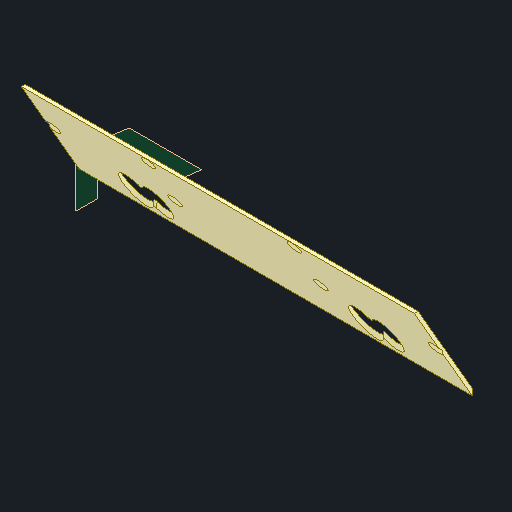
# Autodesk Inventor part: front
Saved by Autodesk Inventor 2023 (Build 270158000, 158)
## iProperties
Created: 2024-05-26
Part Number: front
Material: Nylon 6
Document SubType Name: Modeling
Designer: szymo
Density: 1.12 g/cm^3
Appearance: Nylon 6
Mass: 13.8387 g
Surface Area: 179.282 cm^2
Volume: 12.3559 cm^3
Author: szymo
Autodesk Inventor part; units mm, degrees
ref_plane "YZ Plane" through (0, 0, 0) normal (1, 0, 0) x (0, 1, 0)
ref_plane "XZ Plane" through (0, 0, 0) normal (0, 1, 0) x (-1, 0, 0)
ref_plane "XY Plane" through (0, 0, 0) normal (0, 0, 1) x (1, 0, 0)
ref_plane "Work Plane1" through (-178, 0.5, -3.5) normal (-1, 0, 0) x (0, 0, 1)
sketch "Sketch1" plane through (-178, 0.5, -3.5) normal (-1, 0, 0) x (0, 0, 1)
  line L0 (3.5, 3.5) -> (-1, 3.5) projected
  line L1 (-1, 3.5) -> (-1, -0.5) projected
  line L2 (-1, -0.5) -> (-4.5, -0.5) projected
  line L3 (-4.5, -0.5) -> (-4.5, -14.5) projected
  line L4 (-4.5, -14.5) -> (4.5, -0.5) projected
  line L5 (4.5, -0.5) -> (3.5, -0.5) projected
  line L6 (3.5, -0.5) -> (3.5, 3.5) projected
  circle A0 centre (8.5, 158.5) radius 3 projected
  circle A1 centre (8.5, 158.5) radius 25
  circle A2 centre (13, 116) radius 15 projected
  line L7 (3.5, 3.5) -> (28, 45.9352)
  line L8 (3.5, 0.5) -> (29.7321, 45.9352)
  line L9 (29.7321, 45.9352) -> (28, 45.9352)
  line L10 (28, 45.9352) -> (28, 131) projected
  dimension "d0" = 50
  dimension "d1" = 30
  dimension "d3" = 1.5
  dimension "d4" = 3
  dimension "d5" = 1.7321
  constraints: 6 end point, 2 point on line, 1 centre point, 1 coincident, 1 horizontal, 1 parallel
  measures "d0" diameter of A1
  measures "d1" angle of L7 L6
  measures "d3" distance between parallel lines of L8 L7
  measures "d4" distance of L8.start L0.start
  measures "d5" distance of L7.end L8.end
ref_plane "Work Plane2" through (0, -14, -8) normal (1, 0, 0) x (0, 1, 0)
extrude "Extrusion1" add sketch "Sketch1" against normal up to surface (178 mm away) contours L7 L9 L8 L6
ref_plane "Work Plane3" through (-141.1151, 26.996, 4.2847) normal (0, -0.9925462, 0.1218693) x (1, 0, 0)
sketch "Sketch3" plane through (-141.1151, 26.996, 4.2847) normal (0, -0.9925462, 0.1218693) x (1, 0, 0)
  line L0 (89.3087, 5.4518) -> (89.3087, -5.4534)
  spline S0 degree 3 poles (89.3087, -5.4534) (89.308, -5.5772) (89.3587, -5.6989) (89.4451, -5.7853) (89.4649, -5.8051) (89.4865, -5.823) (89.5096, -5.8388) (89.529, -5.8521) (89.5494, -5.864) (89.5707, -5.8743) (89.5866, -5.882) (89.603, -5.8889) (89.6197, -5.8948) (89.6699, -5.9125) (89.7231, -5.9218) (89.7769, -5.9215) knots 0 0 0 0 0.5 0.5 0.5 0.614375 0.614375 0.614375 0.710781 0.710781 0.710781 0.783086 0.783086 0.783086 1 1 1 1
  line L1 (89.7769, -5.9215) -> (118.6836, -5.9215)
  spline S1 degree 3 poles (118.6836, -5.9215) (118.8077, -5.9222) (118.9296, -5.8713) (119.1025, -5.6977) (119.1524, -5.5758) (119.1517, -5.4518) knots 0 0 0 0 0.5 0.5 1 1 1 1
  line L2 (119.1517, -5.4518) -> (119.1517, 5.4534)
  spline S2 degree 3 poles (119.1517, 5.4534) (119.1524, 5.5775) (119.1015, 5.6994) (118.9279, 5.8723) (118.806, 5.9222) (118.682, 5.9215) knots 0 0 0 0 0.5 0.5 1 1 1 1
  line L3 (118.682, 5.9215) -> (89.7769, 5.9215)
  spline S3 degree 3 poles (89.7769, 5.9215) (89.6527, 5.9222) (89.5308, 5.8713) (89.3579, 5.6977) (89.308, 5.5758) (89.3087, 5.4518) knots 0 0 0 0 0.5 0.5 1 1 1 1
  circle A0 centre (90.8511, -4.3791) radius 0.5
  circle A1 centre (90.8511, 4.3791) radius 0.5
  circle A2 centre (117.6093, 4.3791) radius 0.5
  circle A3 centre (117.6093, -4.3791) radius 0.5
  arc A4 (104.4919, -1.4512) -> (104.4113, -1.5218) centre (104.5073, -1.55) ccw
  arc A5 (104.4113, 1.5218) -> (104.4113, -1.5218) centre (99.2302, 0) ccw
  arc A6 (104.4113, 1.5218) -> (104.4919, 1.4512) centre (104.5073, 1.55) ccw
  arc A7 (104.4919, 1.4512) -> (104.5716, 1.519) centre (104.4765, 1.55) ccw
  arc A8 (104.5716, -1.519) -> (104.5716, 1.519) centre (109.2302, 0) ccw
  arc A9 (104.5716, -1.519) -> (104.4919, -1.4512) centre (104.4765, -1.55) ccw
  line L4 (-14.9215, 5.4518) -> (-14.9215, -5.4534)
  spline S4 degree 3 poles (-14.9215, -5.4534) (-14.9222, -5.5772) (-14.8715, -5.6989) (-14.7851, -5.7853) (-14.7653, -5.8051) (-14.7437, -5.823) (-14.7206, -5.8388) (-14.7012, -5.8521) (-14.6808, -5.864) (-14.6595, -5.8743) (-14.6436, -5.882) (-14.6272, -5.8889) (-14.6105, -5.8948) (-14.5603, -5.9125) (-14.5071, -5.9218) (-14.4534, -5.9215) knots 0 0 0 0 0.5 0.5 0.5 0.614375 0.614375 0.614375 0.710781 0.710781 0.710781 0.783086 0.783086 0.783086 1 1 1 1
  line L5 (-14.4534, -5.9215) -> (14.4534, -5.9215)
  spline S5 degree 3 poles (14.4534, -5.9215) (14.5775, -5.9222) (14.6994, -5.8713) (14.8723, -5.6977) (14.9222, -5.5758) (14.9215, -5.4518) knots 0 0 0 0 0.5 0.5 1 1 1 1
  line L6 (14.9215, -5.4518) -> (14.9215, 5.4534)
  spline S6 degree 3 poles (14.9215, 5.4534) (14.9222, 5.5775) (14.8713, 5.6994) (14.6977, 5.8723) (14.5758, 5.9222) (14.4518, 5.9215) knots 0 0 0 0 0.5 0.5 1 1 1 1
  line L7 (14.4518, 5.9215) -> (-14.4534, 5.9215)
  spline S7 degree 3 poles (-14.4534, 5.9215) (-14.5775, 5.9222) (-14.6994, 5.8713) (-14.8723, 5.6977) (-14.9222, 5.5758) (-14.9215, 5.4518) knots 0 0 0 0 0.5 0.5 1 1 1 1
  circle A10 centre (-13.3791, -4.3791) radius 0.5
  circle A11 centre (-13.3791, 4.3791) radius 0.5
  circle A12 centre (13.3791, 4.3791) radius 0.5
  circle A13 centre (13.3791, -4.3791) radius 0.5
  arc A14 (0.2617, -1.4512) -> (0.1811, -1.5218) centre (0.2771, -1.55) ccw
  arc A15 (0.1811, 1.5218) -> (0.1811, -1.5218) centre (-5, 0) ccw
  arc A16 (0.1811, 1.5218) -> (0.2617, 1.4512) centre (0.2771, 1.55) ccw
  arc A17 (0.2617, 1.4512) -> (0.3414, 1.519) centre (0.2463, 1.55) ccw
  arc A18 (0.3414, -1.519) -> (0.3414, 1.519) centre (5, 0) ccw
  arc A19 (0.3414, -1.519) -> (0.2617, -1.4512) centre (0.2463, -1.55) ccw
  circle A20 centre (99.2302, 0) radius 5.4
  circle A21 centre (109.2302, 0) radius 4.9
  circle A22 centre (-5, 0) radius 5.4
  circle A23 centre (5, 0) radius 4.9
  arc A24 (0.2925, 3.0331) -> (0.2925, -3.0331) centre (-5, 0) ccw
  arc A25 (0.2925, -3.0331) -> (0.2925, 3.0331) centre (5, 0) ccw
  arc A26 (104.5227, -3.0331) -> (104.5227, 3.0331) centre (109.2302, 0) ccw
  arc A27 (104.5227, 3.0331) -> (104.5227, -3.0331) centre (99.2302, 0) ccw
  point P0 (141.1151, -7.5427)
  point P1 (104.4877, 1.2324)
  point P2 (104.4113, 1.5218)
  point P3 (104.4113, -1.5218)
  point P4 (104.4877, -1.2324)
  point P5 (104.5716, -1.519)
  point P6 (104.5716, 1.519)
  point P7 (0.2575, 1.2324)
  point P8 (0.1811, 1.5218)
  point P9 (0.1811, -1.5218)
  point P10 (0.2575, -1.2324)
  point P11 (0.3414, -1.519)
  point P12 (0.3414, 1.519)
  dimension "d19" = 0.7
  dimension "d20" = 0.7
  constraints: 8 centre point, 8 point on circle, 4 coincident, 4 concentric, 2 other
  measures "d19" radial gap between concentric circles of A18 A25
  measures "d20" radial gap between concentric circles of A5 A27
extrude "Extrusion2" cut sketch "Sketch3" along normal up to next contours A27 L3 | L3 A27 A26 L1 | L1 A27 | A4 A20 A21 A9 | A5 A20 A21 | A21 A20 A8 | A6 A7 A21 A20 | A21 A20 | A24 L7 | L7 A24 A25 L5 | L5 A24 | A14 A22 A23 A19 | A15 A22 A23 | A23 A22 A18 | A16 A17 A23 A22 | A23 A22
fillet "Fillet1" radius 1 3 edges at (-140.8226, 17.2803, 8.5334) (-140.8226, 8.5511, 3.4936) (-36.5924, 17.2803, 8.5334)
sketch "Sketch4" plane through (-178, 46.4352, 26.2321) normal (0, -0.5, 0.8660254) x (1, 0, 0)
  circle A0 centre (2.5, -24.2113) radius 1.75
  arc A1 (4, -26.7113) -> (5, -25.7113) centre (4, -25.7113) ccw
  line L0 (5, -22.7113) -> (5, -25.7113)
  arc A2 (5, -22.7113) -> (4, -21.7113) centre (4, -22.7113) ccw
  arc A3 (3, -20.7113) -> (4, -21.7113) centre (4, -20.7113) ccw
  line L1 (3, -2.0207) -> (3, -20.7113)
  ellipse E0 centre (4, -2.0207) end of major axis (4, -0.866) minor radius 1 (4, -0.866) -> (3, -2.0207) ccw
  line L2 (0, -0.866) -> (4, -0.866)
  line L3 (0, -47.5566) -> (0, -0.866)
  line L4 (0, -47.5566) -> (1, -47.5566)
  line L5 (1, -44.0925) -> (1, -47.5566)
  ellipse E1 centre (4, -44.0925) end of major axis (4, -47.5566) minor radius 3 (3, -40.8265) -> (1, -44.0925) ccw
  line L6 (3, -27.7113) -> (3, -40.8265)
  arc A4 (4, -26.7113) -> (3, -27.7113) centre (4, -27.7113) ccw
  circle A5 centre (175.5, -24.2113) radius 1.75
  arc A6 (173, -25.7113) -> (174, -26.7113) centre (174, -25.7113) ccw
  arc A7 (175, -27.7113) -> (174, -26.7113) centre (174, -27.7113) ccw
  line L7 (175, -27.7113) -> (175, -40.8265)
  ellipse E2 centre (174, -44.0925) end of major axis (174, -47.5566) minor radius 3 (177, -44.0925) -> (175, -40.8265) ccw
  line L8 (177, -44.0925) -> (177, -47.5566)
  line L9 (178, -47.5566) -> (177, -47.5566)
  line L10 (178, -47.5566) -> (178, -0.866)
  line L11 (178, -0.866) -> (174, -0.866)
  ellipse E3 centre (174, -2.0207) end of major axis (174, -0.866) minor radius 1 (175, -2.0207) -> (174, -0.866) ccw
  line L12 (175, -2.0207) -> (175, -20.7113)
  arc A8 (174, -21.7113) -> (175, -20.7113) centre (174, -20.7113) ccw
  arc A9 (174, -21.7113) -> (173, -22.7113) centre (174, -22.7113) ccw
  line L13 (173, -22.7113) -> (173, -25.7113)
  circle A10 centre (122, -27.3373) radius 1.75
  circle A11 centre (122, -3.366) radius 1.75
  spline S0 degree 2 poles (123.3222, -34.8373) (123.1151, -34.822) (122.908, -34.8373) knots 0 0 0 1 1 1 weights 1.00008 1.000838 1.00008
  line L14 (124.5, -34.8373) -> (123.3222, -34.8373)
  line L15 (124.5, -0.866) -> (124.5, -34.8373)
  line L16 (124.5, -0.866) -> (119.5, -0.866)
  line L17 (119.5, -0.866) -> (119.5, -34.8373)
  line L18 (122.908, -34.8373) -> (119.5, -34.8373)
  circle A12 centre (56, -27.3373) radius 1.75
  circle A13 centre (56, -3.366) radius 1.75
  spline S1 degree 2 poles (54.6778, -34.8373) (54.8849, -34.822) (55.092, -34.8373) knots 0 0 0 1 1 1 weights 1.00008 1.000838 1.00008
  line L19 (55.092, -34.8373) -> (58.5, -34.8373)
  line L20 (58.5, -0.866) -> (58.5, -34.8373)
  line L21 (53.5, -0.866) -> (58.5, -0.866)
  line L22 (53.5, -0.866) -> (53.5, -34.8373)
  line L23 (53.5, -34.8373) -> (54.6778, -34.8373)
  point P0 (178, -53.3301)
  constraints: 6 coincident, 4 other
hole "Hole2" at (-175.5, 25.4676, 14.1264) at (-122, 22.7604, 12.5634) at (-122, 43.5202, 24.549) at (-56, 22.7604, 12.5634) at (-56, 43.5202, 24.549) at (-2.5, 25.4676, 14.1264) direction (0, 0.5, -0.8660254) diameter 2.9 end through all countersink diameter 6 countersink angle 90 clearance for "Countersunk Flat Head Screw ISO 2009/7046" size "M2.5" standard "ISO"
body "Solid1"
